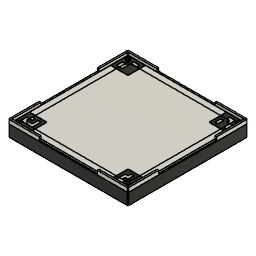
leaf-measurement-box (Autodesk Fusion 360 design; units mm, degrees)
Autodesk Fusion 360 part; units mm, degrees
note: some values were not read from the file. Chosen so that the rebuilt part matches the saved one: which bodies a step acts on. Set by a fixed rule: which sketch regions a step uses; which face or edge a step refers to.
sketch "Sketch1" plane through (0, 0, 0) normal (0, 0, 1) x (1, 0, 0)
  line L0 (0, 0) -> (200, 0)
  line L1 (200, 0) -> (200, 200)
  line L2 (200, 200) -> (0, 200)
  line L3 (0, 200) -> (0, 0)
  line L4 (-2, -3) -> (202, -3)
  line L5 (203, -2) -> (203, 202)
  line L6 (202, 203) -> (-2, 203)
  line L7 (-3, 202) -> (-3, -2)
  arc A0 (-2, 203) -> (-3, 202) centre (-2, 202) ccw
  arc A1 (203, 202) -> (202, 203) centre (202, 202) ccw
  arc A2 (202, -3) -> (203, -2) centre (202, -2) ccw
  arc A3 (-3, -2) -> (-2, -3) centre (-2, -2) ccw
  circle A4 centre (0, 200) radius 1
  circle A5 centre (200, 200) radius 1
  circle A6 centre (200, 0) radius 1
  circle A7 centre (0, 0) radius 1
  line L8 (50, 203) -> (50, 150)
  line L9 (50, 150) -> (-3, 150)
  line L10 (50, 50) -> (-3, 50)
  line L11 (50, 50) -> (50, -3)
  line L12 (150, 50) -> (150, -3)
  line L13 (150, 50) -> (203, 50)
  line L14 (150, 150) -> (150, 203)
  line L15 (150, 150) -> (203, 150)
  dimension "d1" = 200
  dimension "d2" = 200
  dimension "d4" = 1
  dimension "d5" = 2
  dimension "d6" = 2
  dimension "d7" = 2
  dimension "d9" = 2
  constraint horizontal L0
  constraint vertical L1
  constraint horizontal L2
  constraint vertical L3
  constraint coincident L0.start L3.end
  constraint tangent L6 A0
  constraint tangent L7 A0
  constraint tangent L5 A1
  constraint tangent L6 A1
  constraint equal A0 A1
  constraint tangent L4 A2
  constraint tangent L5 A2
  constraint equal A0 A2
  constraint tangent L4 A3
  constraint tangent L7 A3
  constraint equal A0 A3
  constraint coincident L2.end L3.start
  constraint coincident L1.end L2.start
  constraint coincident L0.end L1.start
  constraint coincident L6 L8.start
  constraint perpendicular L6 L8
  constraint coincident L7 L9.end
  constraint perpendicular L7 L9
  constraint coincident L7 L10.end
  constraint perpendicular L7 L10
  constraint coincident L4 L11.end
  constraint perpendicular L4 L11
  constraint coincident L4 L12.end
  constraint perpendicular L4 L12
  constraint coincident L5 L13.end
  constraint perpendicular L5 L13
  constraint coincident L6 L14.end
  constraint perpendicular L6 L14
  constraint coincident L5 L15.end
  constraint perpendicular L5 L15
  measures "d1" distance of L0.start L0.end
  measures "d2" distance of L0.start L2.end
  measures "d4" radius of A0
  measures "d5" diameter of A4
  measures "d6" diameter of A5
  measures "d7" diameter of A6
  measures "d9" diameter of A7
extrude "Extrude1" add sketch "Sketch1" against normal blind 2 makes body 1
extrude "Extrude2" add sketch "Sketch1" along normal blind 5 contours L0 L3 L4 L7 A3 A7 L10 L11 | L0 L1 L4 L5 A2 A6 L12 L13 | L2 L3 L6 L7 A0 A4 L8 L9 | L1 L2 L5 L6 A1 A5 L14 L15 bodies 1
sketch "Sketch2" plane through (0, 0, -2) normal (0, 0, -1) x (1, 0, 0)
  arc A0 (-2, 3) -> (-3, 2) centre (-2, 2) ccw
  line L0 (-3, 2) -> (-3, -202)
  arc A1 (-3, -202) -> (-2, -203) centre (-2, -202) ccw
  line L1 (-2, -203) -> (202, -203)
  arc A2 (202, -203) -> (203, -202) centre (202, -202) ccw
  line L2 (203, -202) -> (203, 2)
  arc A3 (203, 2) -> (202, 3) centre (202, 2) ccw
  line L3 (202, 3) -> (-2, 3)
  line L4 (203, -203) -> (-3, -203)
  line L5 (-3, -203) -> (-3, 3)
  line L6 (-3, 3) -> (203, 3)
  line L7 (203, 3) -> (203, -203)
  line L8 (201, -14) -> (201, -186)
  line L9 (186, -201) -> (14, -201)
  line L10 (-1, -186) -> (-1, -14)
  line L11 (14, 1) -> (186, 1)
  circle A4 centre (195, -195) radius 1.75
  circle A5 centre (195, -195) radius 5
  line L12 (190, -195) -> (190, -197)
  line L13 (195, -190) -> (197, -190)
  circle A6 centre (5, -195) radius 5
  circle A7 centre (5, -195) radius 1.75
  line L14 (10, -195) -> (10, -197)
  line L15 (5, -190) -> (3, -190)
  circle A8 centre (195, -5) radius 5
  circle A9 centre (195, -5) radius 1.75
  line L16 (190, -5) -> (190, -3)
  line L17 (195, -10) -> (197, -10)
  line L18 (10, -5) -> (10, -3)
  line L19 (5, -10) -> (3, -10)
  circle A10 centre (5, -5) radius 5
  circle A11 centre (5, -5) radius 1.75
  arc A12 (10, -197) -> (14, -201) centre (14, -197) ccw
  arc A13 (-1, -186) -> (3, -190) centre (3, -186) ccw
  arc A14 (3, -10) -> (-1, -14) centre (3, -14) ccw
  arc A15 (14, 1) -> (10, -3) centre (14, -3) ccw
  arc A16 (190, -3) -> (186, 1) centre (186, -3) ccw
  arc A17 (201, -14) -> (197, -10) centre (197, -14) ccw
  arc A18 (197, -190) -> (201, -186) centre (197, -186) ccw
  arc A19 (186, -201) -> (190, -197) centre (186, -197) ccw
  dimension "d15" = 3.5
  dimension "d16" = 6
  dimension "d17" = 6
  dimension "d23" = 4
  constraint horizontal L4
  constraint vertical L5
  constraint horizontal L6
  constraint vertical L7
  constraint concentric A4 A5
  constraint coincident A5 L12.start
  constraint tangent A5 L12
  constraint perpendicular L9 L12
  constraint coincident A5 L13.start
  constraint tangent A5 L13
  constraint perpendicular L8 L13
  constraint tangent L14 A12
  constraint tangent L9 A12
  constraint tangent L15 A13
  constraint tangent L10 A13
  constraint equal A12 A13
  constraint tangent L19 A14
  constraint tangent L10 A14
  constraint equal A12 A14
  constraint tangent L18 A15
  constraint tangent L11 A15
  constraint equal A12 A15
  constraint tangent L16 A16
  constraint tangent L11 A16
  constraint equal A12 A16
  constraint tangent L17 A17
  constraint tangent L8 A17
  constraint equal A12 A17
  constraint tangent L8 A18
  constraint tangent L13 A18
  constraint equal A12 A18
  constraint tangent L12 A19
  constraint tangent L9 A19
  constraint equal A12 A19
  measures "d15" diameter of A4
  measures "d16" distance of L9 A4.centre
  measures "d17" distance of L8 A4.centre
  measures "d23" radius of A12
extrude "Extrude3" add sketch "Sketch2" along normal blind 20 separate body contours A0 L0 A1 L1 A2 L2 A3 L3 L4 L5 L6 L7 | A8 | A5 | A10 | A6 makes body 2
sketch "Sketch3" plane through (0, 0, -22) normal (0, 0, -1) x (1, 0, 0)
  circle A0 centre (195, -5) radius 1.75
  line L0 (10, -197) -> (10, -195)
  arc A1 (10, -195) -> (5, -190) centre (5, -195) ccw
  line L1 (5, -190) -> (3, -190)
  arc A2 (-1, -186) -> (3, -190) centre (3, -186) ccw
  line L2 (-1, -186) -> (-1, -14)
  arc A3 (3, -10) -> (-1, -14) centre (3, -14) ccw
  line L3 (3, -10) -> (5, -10)
  arc A4 (5, -10) -> (10, -5) centre (5, -5) ccw
  line L4 (10, -5) -> (10, -3)
  arc A5 (14, 1) -> (10, -3) centre (14, -3) ccw
  line L5 (14, 1) -> (186, 1)
  arc A6 (190, -3) -> (186, 1) centre (186, -3) ccw
  line L6 (190, -3) -> (190, -5)
  arc A7 (190, -5) -> (195, -10) centre (195, -5) ccw
  line L7 (195, -10) -> (197, -10)
  arc A8 (201, -14) -> (197, -10) centre (197, -14) ccw
  line L8 (201, -14) -> (201, -186)
  arc A9 (197, -190) -> (201, -186) centre (197, -186) ccw
  line L9 (197, -190) -> (195, -190)
  arc A10 (195, -190) -> (190, -195) centre (195, -195) ccw
  line L10 (190, -195) -> (190, -197)
  arc A11 (186, -201) -> (190, -197) centre (186, -197) ccw
  line L11 (186, -201) -> (14, -201)
  arc A12 (10, -197) -> (14, -201) centre (14, -197) ccw
  circle A13 centre (5, -195) radius 1.75
  circle A14 centre (5, -5) radius 1.75
  circle A15 centre (195, -195) radius 1.75
  arc A16 (202, -203) -> (203, -202) centre (202, -202) ccw
  line L12 (203, -202) -> (203, 2)
  arc A17 (203, 2) -> (202, 3) centre (202, 2) ccw
  line L13 (202, 3) -> (-2, 3)
  arc A18 (-2, 3) -> (-3, 2) centre (-2, 2) ccw
  line L14 (-3, 2) -> (-3, -202)
  arc A19 (-3, -202) -> (-2, -203) centre (-2, -202) ccw
  line L15 (-2, -203) -> (202, -203)
  line L16 (202, -202) -> (-3, -202)
  line L17 (-3, -202) -> (-3, 3)
  line L18 (-3, 3) -> (202, 3)
  line L19 (202, 3) -> (202, -202)
  constraint horizontal L16
  constraint vertical L17
  constraint horizontal L18
  constraint vertical L19
  constraint coincident A16.centre L16.start
extrude "Extrude4" add sketch "Sketch3" against normal blind 2 contours L0 A1 L1 A2 L2 A3 L3 A4 L4 A5 L5 A6 L6 A7 L7 A8 L8 A9 L9 A10 L10 A11 L11 A12 bodies 2
sketch "Sketch4" plane through (0, 0, -22) normal (0, 0, -1) x (1, 0, 0)
  circle A0 centre (5, -195) radius 1.75
  circle A1 centre (195, -195) radius 1.75
  circle A2 centre (5, -5) radius 1.75
  circle A3 centre (195, -5) radius 1.75
  arc A4 (202, -203) -> (203, -202) centre (202, -202) ccw
  line L0 (203, -202) -> (203, 2)
  arc A5 (203, 2) -> (202, 3) centre (202, 2) ccw
  line L1 (202, 3) -> (-2, 3)
  arc A6 (-2, 3) -> (-3, 2) centre (-2, 2) ccw
  line L2 (-3, 2) -> (-3, -202)
  arc A7 (-3, -202) -> (-2, -203) centre (-2, -202) ccw
  line L3 (-2, -203) -> (202, -203)
  circle A8 centre (5, -5) radius 2.75
  circle A9 centre (195, -5) radius 2.75
  circle A10 centre (195, -195) radius 2.75
  circle A11 centre (5, -195) radius 2.75
  dimension "d28" = 5.5
  dimension "d29" = 5.5
  dimension "d30" = 5.5
  dimension "d31" = 5.5
  constraint concentric A2 A8
  constraint concentric A3 A9
  constraint concentric A1 A10
  constraint concentric A0 A11
  measures "d28" diameter of A8
  measures "d29" diameter of A9
  measures "d30" diameter of A10
  measures "d31" diameter of A11
extrude "Extrude5" cut sketch "Sketch4" against normal blind 3 contours A8 | A9 | A10 | A11 bodies 2
sketch "Sketch5" plane through (0, 0, -2) normal (0, 0, -1) x (1, 0, 0)
  arc A0 (-2, 3) -> (-3, 2) centre (-2, 2) ccw
  line L0 (-3, 2) -> (-3, -202)
  arc A1 (-3, -202) -> (-2, -203) centre (-2, -202) ccw
  line L1 (-2, -203) -> (202, -203)
  arc A2 (202, -203) -> (203, -202) centre (202, -202) ccw
  line L2 (203, -202) -> (203, 2)
  arc A3 (203, 2) -> (202, 3) centre (202, 2) ccw
  line L3 (202, 3) -> (-2, 3)
  line L4 (1.5, 1) -> (199, 1)
  line L5 (201, -1) -> (201, -199)
  line L6 (199, -201) -> (1.5, -201)
  line L7 (-0.5, -199) -> (-0.5, -1)
  arc A4 (199, -201) -> (201, -199) centre (199, -199) ccw
  arc A5 (201, -1) -> (199, 1) centre (199, -1) ccw
  arc A6 (1.5, 1) -> (-0.5, -1) centre (1.5, -1) ccw
  arc A7 (-0.5, -199) -> (1.5, -201) centre (1.5, -199) ccw
  dimension "d34" = 2
  dimension "d55" = 2
  constraint horizontal L4
  constraint vertical L5
  constraint horizontal L6
  constraint vertical L7
  constraint tangent L5 A4
  constraint tangent L6 A4
  constraint tangent L4 A5
  constraint tangent L5 A5
  constraint equal A4 A5
  constraint tangent L4 A6
  constraint tangent L7 A6
  constraint equal A4 A6
  constraint tangent L6 A7
  constraint tangent L7 A7
  measures "d34" radius of A4
  measures "d55" radius of A7
extrude "Extrude6" cut sketch "Sketch5" along normal blind 3.5 contours L4 L5 L6 L7 A4 A5 A6 A7 bodies 2
extrude "Extrude7" add sketch "Sketch5" along normal blind 3 contours L4 L5 L6 L7 A4 A5 A6 A7 bodies 1
extrude "Extrude8" cut sketch "Sketch4" against normal blind 20 contours A0 | A1 | A2 | A3 bodies 1
sketch "Sketch7" plane through (0, 0, 0) normal (0, 0, 1) x (-1, 0, 0)
  line L0 (-200, -50) -> (-203, -50)
  line L1 (-203, -50) -> (-203, -150)
  line L2 (-203, -150) -> (-200, -150)
  line L3 (-200, -150) -> (-200, -199)
  arc A0 (-200, -199) -> (-199, -200) centre (-200, -200) ccw
  line L4 (-199, -200) -> (-150, -200)
  line L5 (-150, -200) -> (-150, -203)
  line L6 (-150, -203) -> (-50, -203)
  line L7 (-50, -203) -> (-50, -200)
  line L8 (-50, -200) -> (-1, -200)
  arc A1 (-1, -200) -> (0, -199) centre (0, -200) ccw
  line L9 (0, -199) -> (0, -150)
  line L10 (0, -150) -> (3, -150)
  line L11 (3, -150) -> (3, -50)
  line L12 (3, -50) -> (0, -50)
  line L13 (0, -50) -> (0, -1)
  arc A2 (0, -1) -> (-1, 0) centre (0, 0) ccw
  line L14 (-1, 0) -> (-50, 0)
  line L15 (-50, 0) -> (-50, 3)
  line L16 (-50, 3) -> (-150, 3)
  line L17 (-150, 3) -> (-150, 0)
  line L18 (-150, 0) -> (-199, 0)
  arc A3 (-199, 0) -> (-200, -1) centre (-200, 0) ccw
  line L19 (-200, -1) -> (-200, -50)
  circle A4 centre (-5, -5) radius 3.25
  circle A5 centre (-5, -195) radius 3.25
  circle A6 centre (-195, -195) radius 3.25
  circle A7 centre (-195, -5) radius 3.25
  dimension "d49" = 6.5
  dimension "d50" = 6.5
  dimension "d51" = 6.5
  dimension "d52" = 6.5
  measures "d49" diameter of A4
  measures "d50" diameter of A5
  measures "d51" diameter of A6
  measures "d52" diameter of A7
extrude "Extrude9" cut sketch "Sketch7" against normal blind 2.5 contours A4 | A5 | A6 | A7 bodies 1
sketch "Sketch8" plane through (0, 0, 0) normal (0, 0, 1) x (-1, 0, 0)
  line L0 (-200, -50) -> (-203, -50)
  line L1 (-203, -50) -> (-203, -150)
  line L2 (-203, -150) -> (-200, -150)
  line L3 (-200, -150) -> (-200, -199)
  arc A0 (-200, -199) -> (-199, -200) centre (-200, -200) ccw
  line L4 (-199, -200) -> (-150, -200)
  line L5 (-150, -200) -> (-150, -203)
  line L6 (-150, -203) -> (-50, -203)
  line L7 (-50, -203) -> (-50, -200)
  line L8 (-50, -200) -> (-1, -200)
  arc A1 (-1, -200) -> (0, -199) centre (0, -200) ccw
  line L9 (0, -199) -> (0, -150)
  line L10 (0, -150) -> (3, -150)
  line L11 (3, -150) -> (3, -50)
  line L12 (3, -50) -> (0, -50)
  line L13 (0, -50) -> (0, -1)
  arc A2 (0, -1) -> (-1, 0) centre (0, 0) ccw
  line L14 (-1, 0) -> (-50, 0)
  line L15 (-50, 0) -> (-50, 3)
  line L16 (-50, 3) -> (-150, 3)
  line L17 (-150, 3) -> (-150, 0)
  line L18 (-150, 0) -> (-199, 0)
  arc A3 (-199, 0) -> (-200, -1) centre (-200, 0) ccw
  line L19 (-200, -1) -> (-200, -50)
  circle A4 centre (-5, -5) radius 3.25
  circle A5 centre (-5, -195) radius 3.25
  circle A6 centre (-195, -5) radius 3.25
  circle A7 centre (-195, -195) radius 3.25
  line L20 (-200, 0) -> (0, 0)
  line L21 (0, 0) -> (0, -200)
  line L22 (0, -200) -> (-200, -200)
  line L23 (-200, -200) -> (-200, 0)
  line L24 (-170, -170) -> (-170, -200)
  line L25 (-170, -170) -> (-200, -170)
  line L26 (-175, -175) -> (-175, -200)
  line L27 (-175, -175) -> (-200, -175)
  line L28 (-180, -180) -> (-200, -180)
  line L29 (-180, -180) -> (-180, -200)
  line L30 (-185, -185) -> (-200, -185)
  line L31 (-185, -185) -> (-185, -200)
  line L32 (-190, -190) -> (-200, -190)
  line L33 (-190, -190) -> (-190, -200)
  line L34 (-200, -195) -> (-195, -195)
  line L35 (-195, -195) -> (-195, -200)
  line L36 (-109.2176, -100) -> (-90, -100)
  line L37 (-100, -90) -> (-100, -115)
  line L38 (-195, -170) -> (-195, -195)
  line L39 (-170, -195) -> (-195, -195)
  line L40 (-190, -170) -> (-190, -190)
  line L41 (-170, -190) -> (-190, -190)
  line L42 (-185, -170) -> (-185, -185)
  line L43 (-170, -185) -> (-185, -185)
  line L44 (-180, -170) -> (-180, -180)
  line L45 (-170, -180) -> (-180, -180)
  line L46 (-175, -170) -> (-175, -175)
  line L47 (-170, -175) -> (-175, -175)
  line L48 (0, -170) -> (0, -200)
  line L49 (0, -170) -> (-30, -170)
  line L50 (-5, -170) -> (-5, -175)
  line L51 (0, -175) -> (-5, -175)
  line L52 (-5, -175) -> (-30, -175)
  line L53 (-5, -175) -> (-5, -200)
  line L54 (0, -180) -> (-10, -180)
  line L55 (-25, -170) -> (-25, -195)
  line L56 (-20, -170) -> (-20, -190)
  line L57 (-15, -170) -> (-15, -185)
  line L58 (-10, -170) -> (-10, -180)
  line L59 (-10, -180) -> (-30, -180)
  line L60 (-15, -185) -> (-30, -185)
  line L61 (-20, -190) -> (-30, -190)
  line L62 (-30, -195) -> (-25, -195)
  line L63 (-25, -195) -> (-25, -200)
  line L64 (-20, -190) -> (-20, -200)
  line L65 (-15, -185) -> (-15, -200)
  line L66 (-10, -180) -> (-10, -200)
  line L67 (0, -195) -> (-25, -195)
  line L68 (0, -190) -> (-20, -190)
  line L69 (0, -185) -> (-15, -185)
  line L70 (-170, 0) -> (-170, -30)
  line L71 (-170, 0) -> (-200, 0)
  line L72 (-175, 0) -> (-175, -5)
  line L73 (-170, -5) -> (-175, -5)
  line L74 (-175, -5) -> (-200, -5)
  line L75 (-175, -5) -> (-175, -30)
  line L76 (-170, -10) -> (-180, -10)
  line L77 (-195, 0) -> (-195, -25)
  line L78 (-190, 0) -> (-190, -20)
  line L79 (-185, 0) -> (-185, -15)
  line L80 (-180, 0) -> (-180, -10)
  line L81 (-180, -10) -> (-200, -10)
  line L82 (-185, -15) -> (-200, -15)
  line L83 (-190, -20) -> (-200, -20)
  line L84 (-200, -25) -> (-195, -25)
  line L85 (-195, -25) -> (-195, -30)
  line L86 (-190, -20) -> (-190, -30)
  line L87 (-185, -15) -> (-185, -30)
  line L88 (-180, -10) -> (-180, -30)
  line L89 (-170, -25) -> (-195, -25)
  line L90 (-170, -20) -> (-190, -20)
  line L91 (-170, -15) -> (-185, -15)
  line L92 (0, 0) -> (0, -30)
  line L93 (0, 0) -> (-30, 0)
  line L94 (-5, 0) -> (-5, -5)
  line L95 (0, -5) -> (-5, -5)
  line L96 (-5, -5) -> (-30, -5)
  line L97 (-5, -5) -> (-5, -30)
  line L98 (0, -10) -> (-10, -10)
  line L99 (-25, 0) -> (-25, -25)
  line L100 (-20, 0) -> (-20, -20)
  line L101 (-15, 0) -> (-15, -15)
  line L102 (-10, 0) -> (-10, -10)
  line L103 (-10, -10) -> (-30, -10)
  line L104 (-15, -15) -> (-30, -15)
  line L105 (-20, -20) -> (-30, -20)
  line L106 (-30, -25) -> (-25, -25)
  line L107 (-25, -25) -> (-25, -30)
  line L108 (-20, -20) -> (-20, -30)
  line L109 (-15, -15) -> (-15, -30)
  line L110 (-10, -10) -> (-10, -30)
  line L111 (0, -25) -> (-25, -25)
  line L112 (0, -20) -> (-20, -20)
  line L113 (0, -15) -> (-15, -15)
  line L114 (-170, -30) -> (-200, -30)
  line L115 (-200, -30) -> (-200, 0)
  line L116 (-200, 0) -> (-170, 0)
  line L117 (-170, 0) -> (-170, -30)
  line L118 (-30, -30) -> (0, -30)
  line L119 (0, -30) -> (0, 0)
  line L120 (0, 0) -> (-30, 0)
  line L121 (-30, 0) -> (-30, -30)
  line L122 (-30, -170) -> (0, -170)
  line L123 (0, -170) -> (0, -200)
  line L124 (0, -200) -> (-30, -200)
  line L125 (-30, -200) -> (-30, -170)
  line L126 (-200, -170) -> (-170, -170)
  line L127 (-170, -170) -> (-170, -200)
  line L128 (-170, -200) -> (-200, -200)
  line L129 (-200, -200) -> (-200, -170)
  line L130 (-200, -200) -> (0, -200)
  line L131 (0, -200) -> (0, 0)
  line L132 (0, 0) -> (-200, 0)
  line L133 (-200, 0) -> (-200, -200)
  dimension "d58" = 170
  dimension "d59" = 170
  constraint horizontal L20
  constraint vertical L21
  constraint horizontal L22
  constraint vertical L23
  constraint coincident A1.centre L21.end
  constraint coincident A3.centre L20.start
  constraint coincident L22 L24.end
  constraint coincident L23 L25.end
  constraint coincident L22 L26.end
  constraint coincident L3 L27.end
  constraint coincident L3 L28.end
  constraint coincident L23 L30.end
  constraint coincident L3 L32.end
  constraint coincident L3 L34.start
  constraint coincident A7.centre L34.end
  constraint coincident L22 L35.end
  constraint vertical L37
  constraint coincident L25 L38.start
  constraint coincident L24 L39.start
  constraint parallel L34 L39
  constraint coincident L25 L40.start
  constraint perpendicular L32 L40
  constraint coincident L24 L41.start
  constraint perpendicular L40 L41
  constraint midpoint L25 L42.start
  constraint perpendicular L30 L42
  constraint midpoint L24 L43.start
  constraint perpendicular L42 L43
  constraint coincident L25 L44.start
  constraint coincident L24 L45.start
  constraint perpendicular L29 L45
  constraint coincident L25 L46.start
  constraint coincident L24 L47.start
  constraint parallel L27 L47
  constraint horizontal L114
  constraint vertical L115
  constraint horizontal L116
  constraint vertical L117
  constraint horizontal L118
  constraint vertical L119
  constraint horizontal L120
  constraint vertical L121
  constraint horizontal L122
  constraint vertical L123
  constraint horizontal L124
  constraint vertical L125
  constraint horizontal L126
  constraint vertical L127
  constraint horizontal L128
  constraint vertical L129
  constraint horizontal L130
  constraint vertical L131
  constraint horizontal L132
  constraint vertical L133
extrude "Extrude10" add sketch "Sketch8" along normal blind 0.3 separate body contours L3 L4 L8 L9 L13 L14 L18 L19 L20 L21 L22 L23 L24 L25 L49 L70 L114 L117 L118 L121 L122 L125 L126 L127 L130 L131 L132 L133 | L27 L28 L38 L40 | L87 L88 L89 L90 | L28 L30 L38 L40 | A6 L74 L77 L78 L81 | L78 L79 L81 L82 | L87 L88 L90 L91 | A6 L74 L77 | L75 L88 L90 L91 | L30 L31 L40 L41 | L26 L27 L44 L45 | L74 L79 L80 L81 | L75 L76 L88 L91 | L31 L33 L39 L41 | L26 L29 L43 L45 | L74 L75 L76 L80 | L29 L31 L39 L41 | L99 L100 L103 L104 | L55 L61 L64 L67 | L100 L101 L103 L104 | L99 L100 L104 L105 | L64 L65 L67 L68 | L101 L103 L110 L113 | L99 L105 L108 L111 | L97 L98 L110 L113 | A5 L53 L66 L67 L68 | L65 L66 L68 L69 | L97 L110 L112 L113 | L109 L110 L111 L112 | A5 L53 L67 | L57 L59 L66 L69 | L53 L54 L66 L69 | L52 L57 L58 L59 | L52 L53 L54 L58 picked at (-192.8444, -5.1542) picked at (-5.1542, -192.8444) makes body 6 at (193.3333, 8.3333, 0) makes body 6 at (188.3333, 11.6667, 0) makes body 6 at (176.6667, 13.3333, 0) makes body 5 at (16.6667, 11.6667, 0) makes body 5 at (13.3333, 21.6667, 0) makes body 4 at (21.6667, 193.3333, 0) makes body 4 at (10, 178.3333, 0) makes body 4 at (8.3333, 191.6667, 0) makes body 7 at (193.3333, 181.6667, 0) makes body 7 at (185, 193.3333, 0) makes body 3 at (123.3333, 76.6667, 0) makes body 8 at (176.6667, 180, 0)
extrude "Extrude11" add sketch "Sketch8" along normal blind 0.3 separate body contours L19 L23 L84 L85 L114 L115 L133 | L19 L23 L77 L83 L84 L115 L133 | L85 L86 L89 L114 | L3 L23 L25 L27 L38 L126 L129 L133 | L19 L23 L77 L82 L83 L115 L133 | L77 L83 L86 L89 | L86 L87 L89 L114 | L3 L23 L27 L28 L38 L129 L133 | L25 L27 L38 L40 L126 | L19 L23 L77 L81 L82 L115 L133 | L77 L78 L82 L83 | L86 L87 L89 L90 | L87 L88 L89 L114 | L3 L23 L28 L30 L38 L129 L133 | L25 L27 L40 L42 L126 | L19 A6 L23 L74 L77 L81 L115 L133 | L77 L78 L81 L82 | L78 L82 L87 L90 | L75 L88 L89 L114 | L3 L23 L30 L32 L38 L129 L133 | L27 L28 L40 L42 | L25 L27 L42 L44 L126 | L18 L19 A6 L20 L23 L71 L74 L77 L115 L116 L132 L133 | L75 L88 L89 L90 | L70 L75 L89 L114 L117 | L3 A7 L23 L32 L34 L38 L129 L133 | L30 L32 L38 L40 | L28 L30 L40 L42 | L27 L28 L42 L44 | L25 L27 L44 L46 L126 | A6 L74 L77 | A6 L74 L77 | L74 L78 L79 L81 | L79 L81 L88 L91 | L70 L75 L89 L90 L117 | L3 L4 A7 L22 L23 L34 L35 L128 L129 L130 L133 | A7 L32 L33 L38 L39 | L28 L29 L42 L43 | L24 L25 L46 L47 L126 L127 | L18 A6 L20 L71 L74 L77 L78 L116 L132 | A6 L74 L77 | L18 L20 L71 L74 L78 L79 L116 L132 | L70 L75 L90 L91 L117 | A7 L34 L35 | A7 L34 L38 | A7 L38 L39 | L29 L31 L41 L43 | L24 L26 L45 L47 L127 | L18 L20 L71 L74 L79 L80 L116 L132 | L70 L75 L76 L91 L117 | A7 L35 L39 | L4 A7 L22 L33 L35 L39 L128 L130 | L4 L22 L31 L33 L39 L128 L130 | L26 L29 L41 L43 | L24 L26 L43 L45 L127 | L18 L20 L71 L72 L74 L80 L116 L132 | L70 L73 L75 L76 L117 | L4 L22 L29 L31 L39 L128 L130 | L26 L29 L39 L41 | L24 L26 L41 L43 L127 | L18 L20 L70 L71 L72 L73 L116 L117 L132 | L4 L22 L26 L29 L39 L128 L130 | L24 L26 L39 L41 L127 | L4 L22 L24 L26 L39 L127 L128 L130 | L14 L20 L93 L96 L99 L120 L121 L132 | L14 L20 L93 L96 L99 L100 L120 L132 | L96 L99 L103 L121 | L8 L22 L62 L63 L124 L125 L130 | L14 L20 L93 L96 L100 L101 L120 L132 | L96 L99 L100 L103 | L99 L103 L104 L121 | L8 L22 L63 L64 L67 L124 L130 | L55 L61 L62 L125 | L14 L20 L93 L96 L101 L102 L120 L132 | L96 L100 L101 L103 | L99 L104 L105 L121 | L8 L22 L64 L65 L67 L124 L130 | L55 L60 L61 L125 | L14 A4 L20 L93 L94 L96 L102 L120 L132 | L96 L101 L102 L103 | L99 L105 L106 L121 | L8 L22 L65 L66 L67 L124 L130 | L55 L56 L60 L61 | L55 L59 L60 L125 | L13 L14 A4 L20 L21 L92 L93 L94 L95 L119 L120 L131 L132 | A4 L96 L97 L98 L102 | L100 L104 L109 L112 | L106 L107 L118 L121 | L8 A5 L22 L53 L66 L67 L124 L130 | L65 L66 L67 L68 | L56 L60 L65 L68 | L55 L56 L59 L60 | L52 L55 L59 L125 | A4 L94 L96 | A4 L94 L95 | A4 L96 L97 | L109 L110 L112 L113 | L108 L109 L111 L112 | L107 L108 L111 L118 | L8 L9 A5 L21 L22 L48 L53 L67 L123 L124 L130 L131 | L56 L57 L59 L60 | L52 L55 L56 L59 | L49 L52 L55 L122 L125 | L13 A4 L21 L92 L95 L97 L98 L119 L131 | A4 L95 L97 | L13 L21 L92 L97 L98 L113 L119 L131 | L108 L109 L111 L118 | A5 L53 L67 | A5 L53 L67 | L53 L66 L68 L69 | L52 L56 L57 L59 | L49 L52 L55 L56 L122 | L13 L21 L92 L97 L112 L113 L119 L131 | L97 L110 L111 L112 | L109 L110 L111 L118 | A5 L53 L67 | L9 A5 L21 L48 L53 L67 L68 L123 L131 | L9 L21 L48 L53 L68 L69 L123 L131 | L49 L52 L56 L57 L122 | L13 L21 L92 L97 L111 L112 L119 L131 | L97 L110 L111 L118 | L9 L21 L48 L53 L54 L69 L123 L131 | L49 L52 L57 L58 L122 | L13 L21 L92 L97 L111 L118 L119 L131 | L9 L21 L48 L51 L53 L54 L123 L131 | L49 L50 L52 L58 L122 | L9 L21 L48 L49 L50 L51 L122 L123 L131 picked at (-197.1556, -5.1542) picked at (-196.2951, -3.2699) picked at (-194.8458, -2.8444) picked at (-2.8444, -195.1542) picked at (-5.1542, -197.1556) picked at (-2.8444, -194.8458) makes body 10 at (191.6667, 23.3333, 0) makes body 10 at (183.3333, 11.6667, 0) makes body 9 at (11.6667, 3.3333, 0) makes body 11 at (23.3333, 178.3333, 0) makes body 12 at (195, 193.3333, 0)
sketch "Sketch9" plane through (0, 0, 0) normal (0, 0, 1) x (-1, 0, 0)
  line L0 (-200, -50) -> (-203, -50)
  line L1 (-203, -50) -> (-203, -150)
  line L2 (-203, -150) -> (-200, -150)
  line L3 (-200, -150) -> (-200, -199)
  arc A0 (-200, -199) -> (-199, -200) centre (-200, -200) ccw
  line L4 (-199, -200) -> (-150, -200)
  line L5 (-150, -200) -> (-150, -203)
  line L6 (-150, -203) -> (-50, -203)
  line L7 (-50, -203) -> (-50, -200)
  line L8 (-50, -200) -> (-1, -200)
  arc A1 (-1, -200) -> (0, -199) centre (0, -200) ccw
  line L9 (0, -199) -> (0, -150)
  line L10 (0, -150) -> (3, -150)
  line L11 (3, -150) -> (3, -50)
  line L12 (3, -50) -> (0, -50)
  line L13 (0, -50) -> (0, -1)
  arc A2 (0, -1) -> (-1, 0) centre (0, 0) ccw
  line L14 (-1, 0) -> (-50, 0)
  line L15 (-50, 0) -> (-50, 3)
  line L16 (-50, 3) -> (-150, 3)
  line L17 (-150, 3) -> (-150, 0)
  line L18 (-150, 0) -> (-199, 0)
  arc A3 (-199, 0) -> (-200, -1) centre (-200, 0) ccw
  line L19 (-200, -1) -> (-200, -50)
  circle A4 centre (-5, -5) radius 3.25
  circle A5 centre (-5, -195) radius 3.25
  circle A6 centre (-195, -5) radius 3.25
  circle A7 centre (-195, -195) radius 3.25
  line L20 (-190, -10) -> (-10, -10)
  line L21 (-10, -10) -> (-10, -190)
  line L22 (-10, -190) -> (-190, -190)
  line L23 (-190, -190) -> (-190, -10)
  constraint horizontal L20
  constraint vertical L21
  constraint horizontal L22
  constraint vertical L23
extrude "Extrude12" cut sketch "Sketch9" against normal blind 10 contours L20 L21 L22 L23 bodies 1
fillet "Fillet1" radius 10 4 edges at (190, 10, -2.5) (10, 10, -2.5) (10, 190, -2.5) (190, 190, -2.5) on bodies 1
sketch "Sketch13" plane through (0, 0, -20) normal (0, 0, 1) x (-1, 0, 0)
  line L0 (-10, -197) -> (-10, -195)
  arc A0 (-5, -190) -> (-10, -195) centre (-5, -195) ccw
  line L1 (-5, -190) -> (-3, -190)
  arc A1 (-3, -190) -> (1, -186) centre (-3, -186) ccw
  line L2 (1, -186) -> (1, -14)
  arc A2 (1, -14) -> (-3, -10) centre (-3, -14) ccw
  line L3 (-3, -10) -> (-5, -10)
  arc A3 (-10, -5) -> (-5, -10) centre (-5, -5) ccw
  line L4 (-10, -5) -> (-10, -3)
  arc A4 (-10, -3) -> (-14, 1) centre (-14, -3) ccw
  line L5 (-14, 1) -> (-186, 1)
  arc A5 (-186, 1) -> (-190, -3) centre (-186, -3) ccw
  line L6 (-190, -3) -> (-190, -5)
  arc A6 (-195, -10) -> (-190, -5) centre (-195, -5) ccw
  line L7 (-195, -10) -> (-197, -10)
  arc A7 (-197, -10) -> (-201, -14) centre (-197, -14) ccw
  line L8 (-201, -14) -> (-201, -186)
  arc A8 (-201, -186) -> (-197, -190) centre (-197, -186) ccw
  line L9 (-197, -190) -> (-195, -190)
  arc A9 (-190, -195) -> (-195, -190) centre (-195, -195) ccw
  line L10 (-190, -195) -> (-190, -197)
  arc A10 (-190, -197) -> (-186, -201) centre (-186, -197) ccw
  line L11 (-186, -201) -> (-14, -201)
  arc A11 (-14, -201) -> (-10, -197) centre (-14, -197) ccw
  line L12 (-26.5, -21) -> (1, -21)
  line L13 (1, -21) -> (1, -10)
  line L14 (1, -10) -> (-26.5, -10)
  line L15 (-26.5, -10) -> (-26.5, -21)
  dimension "d81" = 27.5
  dimension "d82" = 11
  constraint horizontal L12
  constraint vertical L13
  constraint horizontal L14
  constraint vertical L15
  measures "d81" distance of L12.end L12.start
  measures "d82" distance of L14.end L12.start
extrude "Extrude15" cut sketch "Sketch13" along normal blind 18 contours A2 L13 L14 bodies 2
sketch "Sketch10" plane through (-1, 0, 0) normal (1, 0, 0) x (0, 1, 0)
  line L0 (10, -20) -> (186, -20)
  line L1 (186, -20) -> (186, -2)
  line L2 (186, -2) -> (10, -2)
  line L3 (12.5, -15.7) -> (18.5, -15.7)
  line L4 (20, -14.2) -> (20, -13.7)
  line L5 (18.5, -12.2) -> (11, -12.2)
  line L6 (11, -13.7) -> (11, -14.2)
  line L7 (10, -20) -> (19, -20)
  line L8 (12.5, -12.2) -> (19, -12.2)
  line L9 (19, -12.2) -> (19, -4.2)
  line L10 (19, -4.2) -> (11, -4.2)
  line L11 (11, -4.2) -> (11, -12.2)
  arc A0 (12.5, -12.2) -> (11, -13.7) centre (12.5, -13.7) ccw
  arc A1 (11, -14.2) -> (12.5, -15.7) centre (12.5, -14.2) ccw
  arc A2 (18.5, -15.7) -> (20, -14.2) centre (18.5, -14.2) ccw
  arc A3 (20, -13.7) -> (18.5, -12.2) centre (18.5, -13.7) ccw
  line L12 (10, -2) -> (10, -20)
  line L13 (15.5, -15.7) -> (15.5, -16.7114)
  point P0 (11, -15.7)
  point P1 (20, -15.7)
  dimension "d68" = 9
  dimension "d69" = 3.5
  dimension "d71" = 4.3
  dimension "d72" = 8
  dimension "d73" = 1.5
  dimension "d88" = 5.5
  constraint horizontal L3
  constraint vertical L4
  constraint horizontal L5
  constraint vertical L6
  constraint coincident L0 L7.start
  constraint coincident L0 L7.end
  constraint horizontal L8
  constraint vertical L9
  constraint horizontal L10
  constraint vertical L11
  constraint coincident L5.end L6
  constraint coincident L5.end L8
  constraint tangent L6 A0
  constraint tangent L8 A0
  constraint coincident P0 L3
  constraint coincident P0 L6
  constraint tangent L3 A1
  constraint tangent L6 A1
  constraint equal A0 A1
  constraint coincident P1 L3
  constraint coincident P1 L4
  constraint tangent L3 A2
  constraint tangent L4 A2
  constraint equal A0 A2
  constraint tangent L4 A3
  constraint tangent L5 A3
  constraint equal A0 A3
  constraint midpoint L3 L13.start
  constraint perpendicular L3 L13
  measures "d68" distance of P0 P1
  measures "d69" distance of P0 L5.end
  measures "d71" distance of L3 L7
  measures "d72" distance of L5.end L10.end
  measures "d73" radius of A0
  measures "d88" distance of L12 L13
extrude "Extrude13" cut sketch "Sketch10" against normal blind 2 contours L3 L4 L5 L6 L8 A0 A1 A2 A3 bodies 2
move_face "MoveFace1" by (-0.5, 0, 0) 1 faces at (-0.5, 7, -3.1667) on bodies 2
move_face "OffsetFaces2" offset -0.2 2 faces at (-1.6667, 16.5, -12.2) (-1.6667, 14.5, -15.7) on bodies 2
sketch "Sketch14" plane through (-1, 0, 0) normal (1, 0, 0) x (0, 1, 0)
  line L0 (11, -14.4) -> (11, -13.5)
  arc A0 (12.5, -12) -> (11, -13.5) centre (12.5, -13.5) ccw
  line L1 (12.5, -12) -> (18.5, -12)
  arc A1 (20, -13.5) -> (18.5, -12) centre (18.5, -13.5) ccw
  line L2 (20, -13.5) -> (20, -14.4)
  arc A2 (18.5, -15.9) -> (20, -14.4) centre (18.5, -14.4) ccw
  line L3 (18.5, -15.9) -> (12.5, -15.9)
  arc A3 (11, -14.4) -> (12.5, -15.9) centre (12.5, -14.4) ccw
  line L4 (10, -20) -> (186, -20)
  line L5 (186, -20) -> (186, -2)
  line L6 (186, -2) -> (1, -2)
  line L7 (1, -2) -> (1, -5.5)
  line L8 (1, -5.5) -> (10, -5.5)
  line L9 (10.0097, -2) -> (21, -2)
  line L10 (21, -2) -> (21, -20)
  line L11 (21, -20) -> (10.0097, -20)
  line L12 (10.0097, -20) -> (10.0097, -2)
  line L13 (11, -14.4) -> (21, -14.4)
  line L14 (10, -5.5) -> (10, -20)
  line L15 (10, -7) -> (21, -7)
  dimension "d89" = 1
  constraint horizontal L9
  constraint vertical L10
  constraint horizontal L11
  constraint vertical L12
  constraint coincident L4 L10.end
  constraint coincident L6 L9.start
  constraint coincident L0.start A3.start
  constraint coincident L10 L13.end
  constraint perpendicular L10 L13
  constraint coincident L14 L15.start
  constraint coincident L10 L15.end
  constraint perpendicular L10 L15
  measures "d89" distance of L2 L10
extrude "Extrude16" cut sketch "Sketch14" against normal blind 0.7 contours L4 L10 L11 L12 L15 bodies 2
sketch "Sketch15" plane through (0, 0, -2) normal (0, 0, 1) x (-1, 0, 0)
  line L0 (1, -1) -> (1, -186)
  arc A0 (0.5, -187.9365) -> (1, -186) centre (-3, -186) ccw
  line L1 (0.5, -187.9365) -> (0.5, -199)
  arc A1 (-1.5, -201) -> (0.5, -199) centre (-1.5, -199) ccw
  line L2 (-1.5, -201) -> (-199, -201)
  arc A2 (-201, -199) -> (-199, -201) centre (-199, -199) ccw
  line L3 (-201, -199) -> (-201, -1)
  arc A3 (-199, 1) -> (-201, -1) centre (-199, -1) ccw
  line L4 (-199, 1) -> (-1, 1)
  arc A4 (1, -1) -> (-1, 1) centre (-1, -1) ccw
  line L5 (2, 3) -> (-202, 3)
  arc A5 (-202, 3) -> (-203, 2) centre (-202, 2) ccw
  line L6 (-203, 2) -> (-203, -202)
  arc A6 (-203, -202) -> (-202, -203) centre (-202, -202) ccw
  line L7 (-202, -203) -> (2, -203)
  arc A7 (2, -203) -> (3, -202) centre (2, -202) ccw
  line L8 (3, -202) -> (3, 2)
  arc A8 (3, 2) -> (2, 3) centre (2, 2) ccw
  line L9 (5, 5) -> (-30, 5)
  line L10 (-30, 5) -> (-30, -25)
  line L11 (-30, -25) -> (5, -25)
  line L12 (5, -25) -> (5, 5)
  constraint horizontal L9
  constraint vertical L10
  constraint horizontal L11
  constraint vertical L12
